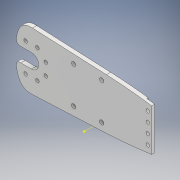
# Autodesk Inventor part: new_side_u106_long_design
Saved by Autodesk Inventor 2018 (Build 220112000, 112)
## iProperties
Created: 2016-12-19
Part Number: new_side_u106_long_design
Material: Aluminum 2014-T4
Document SubType Name: Modeling
Designer: steve
Density: 2.8 g/cm^3
Appearance: Satin
Mass: 27.2523 g
Surface Area: 77.5183 cm^2
Volume: 9.73296 cm^3
Vendor: Rhoban
Author: steve
Autodesk Inventor part; units mm, degrees
ref_plane "YZ Plane" through (0, 0, 0) normal (1, 0, 0) x (0, 1, 0)
ref_plane "XZ Plane" through (0, 0, 0) normal (0, 1, 0) x (-1, 0, 0)
ref_plane "XY Plane" through (0, 0, 0) normal (0, 0, 1) x (1, 0, 0)
sketch "Sketch1" plane through (0, 0, 0) normal (0, 1, 0) x (-1, 0, 0)
  line L0 (-85.5, 15) -> (0, 15) construction
  line L1 (16, 15) -> (16, -15) construction
  line L2 (16, -15) -> (0, -15) construction
  line L3 (-85.5, -15) -> (-85.5, 15)
  line L4 (16, 0) -> (-42.75, 0) construction
  line L5 (-28.4, 0) -> (23.4, 0) construction
  circle A0 centre (0, 0) radius 11 construction
  line L6 (11, 12.5) -> (11, -13.4099) construction
  circle A1 centre (0, 0) radius 5.05 construction
  line L7 (0, 5.05) -> (7.55, 5.05) construction
  line L8 (0, -5.05) -> (7.55, -5.05) construction
  line L9 (16, 15) -> (16, 5) construction
  line L10 (16, -5) -> (16, -15) construction
  arc A2 (0, 5.05) -> (0, -5.05) centre (0, 0) ccw
  circle A3 centre (0, 0) radius 15 construction
  arc A4 (0, -15) -> (14.1421, -5) centre (0, 0) ccw construction
  arc A5 (14.1421, 5) -> (0, 15) centre (0, 0) ccw construction
  line L11 (0, -15) -> (-85.5, -15) construction
  line L12 (0, 15) -> (16, 15) construction
  arc A6 (11, -8.6603) -> (11, 8.6603) centre (0, 0) ccw construction
  line L13 (-3, -24.7441) -> (-3, 29.6212) construction
  arc A7 (-3, -13.6748) -> (7.55, -11.7897) centre (0, 0) ccw
  line L14 (7.55, 5.05) -> (0, 5.05)
  line L15 (-15, -18.6523) -> (-15, 18.2394) construction
  line L16 (-85.5, -15) -> (-15, -15)
  line L17 (-85.5, 15) -> (-15, 15)
  spline S0 degree 4 poles (-3, -13.6748) (-4.5129, -13.3429) (-7.4407, -12.2328) (-10.459, -15) (-13.4863, -15) (-15, -15) knots 0 0 0 0 0 0.5 1 1 1 1 1
  spline S1 degree 4 poles (-3, 13.6748) (-4.5129, 13.3429) (-7.4407, 12.2328) (-10.459, 15) (-13.4863, 15) (-15, 15) knots 0 0 0 0 0 0.5 1 1 1 1 1
  line L18 (5.05, -20.2789) -> (5.05, 16.2453) construction
  line L19 (7.55, -11.7897) -> (7.55, -5.05)
  line L20 (7.55, 5.05) -> (7.55, 11.7897)
  line L21 (7.55, -5.05) -> (11, -5.05) construction
  line L22 (7.55, 5.05) -> (9.7723, 5.05) construction
  arc A8 (7.55, 11.7897) -> (7.55, -11.7897) centre (0, 0) ccw construction
  arc A9 (7.55, 11.7897) -> (-3, 13.6748) centre (0, 0) ccw
  line L23 (0, -5.05) -> (7.55, -5.05)
  line L24 (0, -35.9242) -> (0, 40.5454) construction
  line L25 (45.18, 0) -> (-107.28, 0) projected
  line L26 (-42.75, 0) -> (-85.5, 0) construction
  line L27 (-85.5, 0) -> (-44.5655, 0)
  line L28 (-85.5, 0) -> (-37.398, 0)
  line L29 (-37.398, 0) -> (-37.398, -25) construction
  line L30 (-85.5, 15) -> (-85.5, -25) construction
  line L31 (-85.5, -25) -> (-37.398, -25) construction
  point P0 (13.0767, -5)
  point P1 (13.0767, 5)
  dimension "d1" = 22
  dimension "d0" = 30
  dimension "d2" = 85.5
  dimension "d3" = 10.1
  dimension "d4" = 30
  dimension "d5" = 28
  dimension "d6" = 15
  dimension "d7" = 12
  dimension "d8" = 2.5
  dimension "d76" = 48.102
  dimension "d77" = 40
  constraints: 60 end point, 22 point on circle, 17 point on line, 9 centre point, 8 coincident, 8 collinear, 7 perpendicular, 6 horizontal, 6 vertical, 5 parallel, 4 tangent, 2 midpoint, 8 other
  measures "d0" distance of L9.start L2.start
  measures "d2" distance from line of point (0, 0) L3
  measures "d3" diameter of A1
  measures "d4" diameter of A3
  measures "d5" diameter of A6
  measures "d6" distance from line of L15 point (0, 0)
  measures "d7" distance between parallel lines of L13 L15
  measures "d8" distance between parallel lines of L19 L18
  measures "d76" distance of L30.end L29.end
  measures "d77" distance of L0.start L30.end
extrude "Extrusion1" add sketch "Sketch1" along normal blind 3
sketch "Sketch2" plane through (0, 3, 0) normal (0, 1, 0) x (1, 0, 0)
  circle A0 centre (0, 0) radius 11 construction
  line L0 (-30.3, 0) -> (104.8, 0) construction
  line L1 (0, 21) -> (0, -21) construction
  line L2 (0, 0) -> (-4.2095, -10.1627) construction
  point P0 (-4.2095, -10.1627)
  point P1 (4.2095, -10.1627)
  point P2 (10.1627, -4.2095)
  point P3 (10.1627, 4.2095)
  point P4 (4.2095, 10.1627)
  point P5 (-4.2095, 10.1627)
  dimension "d19" = 22
  dimension "d20" = 225
  dimension "d78" = 22.5
  constraints: 3 coincident, 2 end point, 2 point on circle, 1 centre point, 6 other
  measures "d19" diameter of A0
  measures "d78" angle of L2 L1
hole "Hole1" at (-4.2095, 3, 10.1627) at (-4.2095, 3, -10.1627) at (4.2095, 3, -10.1627) at (10.1627, 3, -4.2095) at (10.1627, 3, 4.2095) at (4.2095, 3, 10.1627) direction (0, -1, 0) diameter 2.5 end through all
sketch "Sketch3" plane through (0, 3, 0) normal (0, 1, 0) x (1, 0, 0)
  circle A0 centre (-4.2095, -10.1627) radius 1.25 construction
  circle A1 centre (4.2095, -10.1627) radius 1.25 construction
  circle A2 centre (10.1627, -4.2095) radius 1.25 construction
  circle A3 centre (10.1627, 4.2095) radius 1.25 construction
  circle A4 centre (4.2095, 10.1627) radius 1.25 construction
  circle A5 centre (-4.2095, 10.1627) radius 1.25 construction
  point P0 (0, 0)
sketch "Sketch4" plane through (0, 3, 0) normal (0, 1, 0) x (1, 0, 0)
  line L0 (82.75, -15) -> (82.75, 10.5) construction
  line L1 (85.5, -15) -> (85.5, 15) construction
  line L2 (15, -15) -> (85.5, -15) construction
  point P0 (0, 0)
  point P1 (82.75, -10.5)
  point P2 (82.75, -3.5)
  point P3 (82.75, 3.5)
  dimension "d29" = 2.75
  dimension "d30" = 4.5
  dimension "d33" = 7
  constraints: 2 end point, 2 point on line, 2 vertical, 1 coincident, 3 other
  measures "d29" distance between parallel lines of L1 L0
  measures "d30" distance from line of L2 point (82.75, -10.5)
  measures "d33" distance of point (82.75, -10.5) point (82.75, -3.5)
hole "Hole2" at (82.75, 3, 10.5) at (82.75, 3, 3.5) at (82.75, 3, -3.5) at (82.75, 3, -10.5) direction (0, -1, 0) diameter 2.5 end through all
sketch "Sketch6" plane through (0, 3, 0) normal (0, 1, 0) x (1, 0, 0)
  line L0 (15, -15) -> (85.5, -15) projected
  line L1 (80, -15) -> (80, 15)
  line L2 (80, 15) -> (85.5, 15)
  line L3 (85.5, 15) -> (85.5, -15)
  line L4 (85.5, -15) -> (85.5, -15)
  line L5 (80, -15) -> (80, -15)
  line L6 (80, -15) -> (85.5, -15)
  line L7 (85.5, 15) -> (15, 15) projected
  line L8 (85.5, -15) -> (85.5, 15) projected
  point P0 (0, 0)
  dimension "d47" = 5.5
  constraints: 12 end point, 3 collinear, 2 vertical, 1 parallel, 1 perpendicular, 1 point on line
  measures "d47" distance between parallel lines of L1 L3
extrude "Extrusion2" cut sketch "Sketch6" against normal blind 1
sketch "Sketch7" plane through (0, 3, 0) normal (0, 1, 0) x (1, 0, 0)
  line L0 (-7.55, -13) -> (80, -13) construction
  line L1 (-7.55, 13) -> (80, 13) construction
  line L2 (80, -15) -> (80, 15) construction
  line L3 (80, 15) -> (15, 15) construction
  arc A0 (3, 13.6748) -> (-7.55, 11.7897) centre (0, 0) ccw construction
  line L4 (-7.55, 11.7897) -> (-7.55, 5.05) construction
  line L5 (-7.55, 5.05) -> (0, 5.05) construction
  arc A1 (0, -5.05) -> (0, 5.05) centre (0, 0) ccw construction
  line L6 (0, -5.05) -> (-7.55, -5.05) construction
  line L7 (-7.55, -5.05) -> (-7.55, -11.7897) construction
  arc A2 (-7.55, -11.7897) -> (3, -13.6748) centre (0, 0) ccw construction
  line L8 (15, -15) -> (80, -15) construction
  circle A3 centre (10.1627, -4.2095) radius 1.25 construction
  circle A4 centre (4.2095, 10.1627) radius 1.25 construction
  circle A5 centre (-4.2095, -10.1627) radius 1.25 construction
  circle A6 centre (-4.2095, 10.1627) radius 1.25 construction
  circle A7 centre (10.1627, 4.2095) radius 1.25 construction
  circle A8 centre (4.2095, -10.1627) radius 1.25 construction
  line L9 (30, -13) -> (30, 13) construction
  line L10 (50, -13) -> (50, 13) construction
  line L11 (-7.55, -5.05) -> (-7.55, -11.7897) projected
  line L12 (-7.55, 11.7897) -> (-7.55, 5.05) projected
  line L13 (80, -15) -> (80, 15) projected
  dimension "d50" = 2
  dimension "d51" = 2
  dimension "d52" = 30
  dimension "d53" = 20
  constraints: 12 end point, 8 point on line, 2 horizontal, 2 vertical, 2 other
  measures "d50" distance between parallel lines of L8 L0
  measures "d51" distance between parallel lines of L3 L1
  measures "d52" distance from line of L9 point (0, 0)
  measures "d53" distance between parallel lines of L10 L9
hole "Hole3" at (30, 3, 13) at (30, 3, -13) at (50, 3, 13) at (50, 3, -13) direction (0, -1, 0) diameter 3 end through all
sketch "Sketch9" plane through (0, 0, 0) normal (0, -1, 0) x (1, 0, 0)
  circle A0 centre (50, 13) radius 1.5 projected
  circle A1 centre (30, 13) radius 1.5 projected
  circle A2 centre (30, -13) radius 1.5 projected
  circle A3 centre (50, -13) radius 1.5 projected
  circle A4 centre (82.75, -3.5) radius 1.25 projected
  circle A5 centre (82.75, 10.5) radius 1.25 projected
  circle A6 centre (82.75, 3.5) radius 1.25 projected
  circle A7 centre (82.75, -10.5) radius 1.25 projected
  circle A8 centre (10.1627, 4.2095) radius 1.25 projected
  circle A9 centre (4.2095, -10.1627) radius 1.25 projected
  circle A10 centre (-4.2095, 10.1627) radius 1.25 projected
  circle A11 centre (-4.2095, -10.1627) radius 1.25 projected
  circle A12 centre (10.1627, -4.2095) radius 1.25 projected
  circle A13 centre (4.2095, 10.1627) radius 1.25 projected
  line L0 (85.5, -15) -> (85.5, 15) projected
  line L1 (85.5, 15) -> (15, 15) projected
  spline S0 degree 4 poles (15, 15) (13.4863, 15) (10.459, 15) (7.4407, 12.2328) (4.5129, 13.3429) (3, 13.6748) knots 0 0 0 0 0 0.5 1 1 1 1 1 projected
  arc A14 (3, 13.6748) -> (-7.55, 11.7897) centre (0, 0) ccw projected
  line L2 (-7.55, 11.7897) -> (-7.55, 5.05) projected
  line L3 (-7.55, 5.05) -> (0, 5.05) projected
  arc A15 (0, -5.05) -> (0, 5.05) centre (0, 0) ccw projected
  line L4 (0, -5.05) -> (-7.55, -5.05) projected
  line L5 (-7.55, -5.05) -> (-7.55, -11.7897) projected
  arc A16 (-7.55, -11.7897) -> (3, -13.6748) centre (0, 0) ccw projected
  spline S1 degree 4 poles (3, -13.6748) (4.5129, -13.3429) (7.4407, -12.2328) (10.459, -15) (13.4863, -15) (15, -15) knots 0 0 0 0 0 0.5 1 1 1 1 1 projected
  line L6 (15, -15) -> (85.5, -15) projected
  line L7 (-33.5183, 0) -> (105.3801, 0) construction
  line L8 (53.3261, -18.0641) -> (0.6359, -20.4888)
  spline S2 degree 4 poles (0.6359, -20.4888) (-4.0309, -20.7036) (-10.0323, -18.8785) (-12.1817, -5.2973) (-9.7602, -5.05) (-7.55, -5.05) knots 0 0 0 0 0 0.549784 1 1 1 1 1
  line L9 (15, -15) -> (85.5, -15) projected
  arc A17 (53.3261, -18.0641) -> (85.5, -15) centre (38.1482, 311.7572) ccw
  line L10 (85.5, 15) -> (15, 15) projected
  line L11 (-11.2901, -5.05) -> (-3.8099, -5.05) construction
  arc A18 (-4.5618, -5.1264) -> (-10.5382, -5.1264) centre (-7.55, -63.5612) ccw construction
  line L12 (-7.55, -5.05) -> (0, -5.05) projected
  line L13 (3.8326, -20.3417) -> (-2.5609, -20.6359) construction
  arc A19 (-1.9144, -20.4771) -> (3.1743, -20.2429) centre (-0.5233, 4.7003) ccw construction
  line L14 (0, 5.05) -> (-7.55, 5.05) projected
  spline S3 degree 4 poles (0.6359, 20.4888) (-4.0309, 20.7036) (-10.0323, 18.8785) (-12.1817, 5.2973) (-9.7602, 5.05) (-7.55, 5.05) knots 0 0 0 0 0 0.549784 1 1 1 1 1
  line L15 (53.3261, 18.0641) -> (0.6359, 20.4888)
  arc A20 (85.5, 15) -> (53.3261, 18.0641) centre (38.1482, -311.7572) ccw
  line L16 (-11.2901, 5.05) -> (-3.8099, 5.05) construction
  arc A21 (-10.5382, 5.1264) -> (-4.5618, 5.1264) centre (-7.55, 63.5612) ccw construction
  line L17 (3.8326, 20.3417) -> (-2.5609, 20.6359) construction
  arc A22 (3.1743, 20.2429) -> (-1.9144, 20.4771) centre (-0.5233, -4.7003) ccw construction
  point P0 (-8.9748, -15.1711)
  point P1 (-10.2976, -6.0407)
  point P2 (-8.9748, 15.1711)
  point P3 (-10.2976, 6.0407)
  constraints: 15 symmetric about line, 12 end point, 8 point on circle, 6 centre point, 6 midpoint, 2 collinear, 2 horizontal, 1 tangent, 19 other
extrude "Extrusion6" add sketch "Sketch9" against normal blind 3 contours A17 L8 S2 L5 A16 S1 L6 | L1 S0 A14 L2 S3 L15 A20
sketch "Sketch8" plane through (0, 3, 0) normal (0, 1, 0) x (1, 0, 0)
  line L0 (-26.16, 0) -> (104.11, 0) construction
  line L1 (80, -15) -> (80, 15) construction
  line L2 (77, -1.55) -> (80, -1.55)
  line L3 (80, -1.55) -> (80, 1.55)
  line L4 (80, 1.55) -> (77, 1.55)
  line L5 (77, 1.55) -> (77, -1.55) construction
  line L6 (77, -1.55) -> (80, 1.55) construction
  line L7 (80, -1.55) -> (77, 1.55) construction
  arc A0 (77, 1.55) -> (77, -1.55) centre (77, 0) ccw
  point P0 (0, 0)
  point P1 (78.5, 0)
  dimension "d61" = 3
  dimension "d62" = 3.1
  constraints: 12 end point, 3 midpoint, 2 parallel, 2 point on circle, 2 point on line, 1 centre point, 1 horizontal, 1 perpendicular
  measures "d61" distance of L3.end L4.end
  measures "d62" distance of L4.end L2.start
extrude "Extrusion3" cut sketch "Sketch8" against normal blind 1
sketch "Sketch10" plane through (0, 2, 0) normal (0, 1, 0) x (1, 0, 0)
  circle A0 centre (82.75, 3.5) radius 1.25 projected
  circle A1 centre (82.75, -10.5) radius 1.25 projected
  circle A2 centre (82.75, -3.5) radius 1.25 projected
  circle A3 centre (82.75, 10.5) radius 1.25 projected
  line L0 (85.5, 15) -> (85.5, -15) projected
  line L1 (80, 15) -> (85.5, 15) projected
  line L2 (80, 1.55) -> (80, 15) projected
  line L3 (77, 1.55) -> (80, 1.55) projected
  arc A4 (77, 1.55) -> (77, -1.55) centre (77, 0) ccw projected
  line L4 (80, -1.55) -> (77, -1.55) projected
  line L5 (80, -15) -> (80, -1.55) projected
  line L6 (85.5, -15) -> (80, -15) projected
  line L7 (80, -15) -> (80, -15.7499)
  line L8 (80, -15.7499) -> (85.5, -15.7499)
  line L9 (85.5, 15) -> (85.5, -15) projected
  line L10 (85.5, -15.7499) -> (85.5, -15)
  line L11 (-31.7181, 0) -> (105.0363, 0) construction
  line L12 (80, 15) -> (80, 15.7499)
  line L13 (80, 15.7499) -> (85.5, 15.7499)
  line L14 (85.5, 15.7499) -> (85.5, 15)
  arc A5 (53.3261, -18.0641) -> (85.5, -15) centre (38.1482, 311.7572) ccw projected
  point P0 (0, 0)
  constraints: 12 end point, 2 symmetric about line, 1 collinear, 1 perpendicular, 1 point on circle, 1 vertical
extrude "Extrusion7" cut sketch "Sketch10" along normal blind 1 contours L1 L12 L13 L14 | A5 L7 L6 | L10 L8 A5
ref_plane "Work Plane1" through (-10.6877, 1.5, -8.1148) normal (-1, 0, 0) x (0, -1, 0)
equation "\"d3\" = d12 + diameter_tol"
equation "\"d19\" = d21"
equation "\"d29\" = hole_2_bottom"
equation "\"d47\" = border_thickness"
equation "\"d10\" = 22"
equation "\"d12\" = 10"
equation "\"d14\" = 2 * d13"
equation "\"base_width\" = 6.25"
equation "\"d21\" = 22"
equation "\"diameter_tol\" = 0.1"
equation "\"border_thickness\" = 5.5"
equation "\"hole_2_bottom\" = 2.75"
equation "\"d13\" = 3"
body "Solid1"
